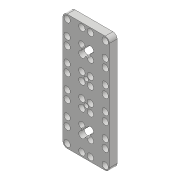
# Autodesk Inventor part: Battery_Cover
Saved by Autodesk Inventor 2018 (Build 220112000, 112)
## iProperties
Created: 2019-09-17
Part Number: Battery_Cover
Material: Generic
Document SubType Name: Modeling
Designer: Clevo
Density: 1 g/cm^3
Appearance: Default
Author: Clevo
Autodesk Inventor part; units mm, degrees
ref_plane "YZ Plane" through (0, 0, 0) normal (1, 0, 0) x (0, 1, 0)
ref_plane "XZ Plane" through (0, 0, 0) normal (0, 1, 0) x (-1, 0, 0)
ref_plane "XY Plane" through (0, 0, 0) normal (0, 0, 1) x (1, 0, 0)
sketch "Sketch1" plane through (0, 0, 0) normal (0, 1, 0) x (-1, 0, 0)
  line L0 (-22, -55) -> (22, -55)
  line L1 (22, -55) -> (22, 55)
  line L2 (22, 55) -> (-22, 55)
  line L3 (-22, 55) -> (-22, -55)
  line L4 (-22, -55) -> (22, 55) construction
  line L5 (22, -55) -> (-22, 55) construction
  point P0 (0, 0)
  dimension "d0" = 110
  dimension "d1" = 44
  constraints: 12 end point, 2 midpoint, 2 parallel, 1 horizontal, 1 perpendicular
  measures "d0" distance of L0.end L1.end
  measures "d1" distance of L1.end L2.end
extrude "Extrusion1" add sketch "Sketch1" along normal blind 7.3
sketch "Sketch2" plane through (0, 7.3, 0) normal (0, 1, 0) x (1, 0, 0)
  line L0 (22, 55) -> (-22, 55) projected
  line L1 (-22, 55) -> (-22, -55) projected
  line L2 (-22, -55) -> (22, -55) projected
  line L3 (22, -55) -> (22, 55) projected
  line L4 (0, -33) -> (-22, -33)
  line L5 (-22, -33) -> (-22, -55)
  line L6 (-22, -55) -> (0, -55)
  line L7 (0, -55) -> (0, -33)
  line L8 (0, -33) -> (-22, -55) construction
  line L9 (-22, -33) -> (0, -55) construction
  line L10 (-4, -37) -> (-18, -37)
  line L11 (-18, -37) -> (-18, -51)
  line L12 (-18, -51) -> (-4, -51)
  line L13 (-4, -51) -> (-4, -37)
  line L14 (-4, -37) -> (-18, -51) construction
  line L15 (-18, -37) -> (-4, -51) construction
  circle A0 centre (-18, -51) radius 3
  line L16 (-22, 55) -> (-22, -55) projected
  circle A1 centre (-18, -37) radius 3
  circle A2 centre (-4, -51) radius 3
  circle A3 centre (-4, -37) radius 3
  circle A4 centre (-11, -44) radius 3.75
  point P0 (0, 0)
  dimension "d4" = 22
  dimension "d5" = 22
  dimension "d6" = 14
  dimension "d7" = 7.5
  dimension "d12" = 6
  dimension "d13" = 6
  dimension "d14" = 6
  dimension "d15" = 6
  constraints: 24 end point, 5 centre point, 5 coincident, 4 midpoint, 4 parallel, 2 horizontal, 2 perpendicular, 1 point on line
  measures "d4" distance of L4.start L4.end
  measures "d5" distance of L6.end L4.start
  measures "d6" distance of L11.end L12.end
  measures "d7" diameter of A4
  measures "d12" diameter of A0
  measures "d13" diameter of A1
  measures "d14" diameter of A3
  measures "d15" diameter of A2
extrude "Extrusion2" cut sketch "Sketch2" against normal blind 7 contours A1 L11 L10 | L10 L11 A1 | A3 L13 L10 | L10 L13 A3 | A0 L12 L11 | L11 L12 A0 | A2 L12 L13 | L13 L12 A2 | A4
sketch "Sketch3" plane through (0, 0.3, 0) normal (0, 1, 0) x (1, 0, 0)
  circle A0 centre (-18, -51) radius 3 projected
  circle A1 centre (-18, -37) radius 3 projected
  circle A2 centre (-4, -51) radius 3 projected
  circle A3 centre (-4, -37) radius 3 projected
  point P0 (0, 0)
extrude "Extrusion3" cut sketch "Sketch3" against normal through all
pattern_linear "Rectangular Pattern1" count 5 spacing 22 along (0, 0, -1) count 2 spacing 22 along (1, 0, 0) of "Extrusion2", "Extrusion3"
sketch "Sketch4" plane through (0, 7.3, 0) normal (0, 1, 0) x (1, 0, 0)
  circle A0 centre (18, 51) radius 3 projected
  circle A1 centre (4, 51) radius 3 projected
  circle A2 centre (4, 37) radius 3 projected
  circle A3 centre (18, 37) radius 3 projected
  circle A4 centre (11, 44) radius 3.75 projected
  circle A5 centre (18, 29) radius 3 projected
  circle A6 centre (4, 29) radius 3 projected
  circle A7 centre (4, 15) radius 3 projected
  circle A8 centre (18, 15) radius 3 projected
  circle A9 centre (11, 22) radius 3.75 projected
  circle A10 centre (18, 7) radius 3 projected
  circle A11 centre (4, 7) radius 3 projected
  circle A12 centre (4, -7) radius 3 projected
  circle A13 centre (18, -7) radius 3 projected
  circle A14 centre (11, 0) radius 3.75 projected
  circle A15 centre (18, -15) radius 3 projected
  circle A16 centre (4, -15) radius 3 projected
  circle A17 centre (4, -29) radius 3 projected
  circle A18 centre (18, -29) radius 3 projected
  circle A19 centre (11, -22) radius 3.75 projected
  circle A20 centre (18, -37) radius 3 projected
  circle A21 centre (4, -37) radius 3 projected
  circle A22 centre (4, -51) radius 3 projected
  circle A23 centre (18, -51) radius 3 projected
  circle A24 centre (11, -44) radius 3.75 projected
  circle A25 centre (-4, 51) radius 3 projected
  circle A26 centre (-18, 51) radius 3 projected
  circle A27 centre (-18, 37) radius 3 projected
  circle A28 centre (-4, 37) radius 3 projected
  circle A29 centre (-11, 44) radius 3.75 projected
  circle A30 centre (-4, 29) radius 3 projected
  circle A31 centre (-18, 29) radius 3 projected
  circle A32 centre (-18, 15) radius 3 projected
  circle A33 centre (-4, 15) radius 3 projected
  circle A34 centre (-11, 22) radius 3.75 projected
  circle A35 centre (-4, 7) radius 3 projected
  circle A36 centre (-18, 7) radius 3 projected
  circle A37 centre (-18, -7) radius 3 projected
  circle A38 centre (-4, -7) radius 3 projected
  circle A39 centre (-11, 0) radius 3.75 projected
  circle A40 centre (-4, -15) radius 3 projected
  circle A41 centre (-18, -15) radius 3 projected
  circle A42 centre (-18, -29) radius 3 projected
  circle A43 centre (-4, -29) radius 3 projected
  circle A44 centre (-11, -22) radius 3.75 projected
  circle A45 centre (-11, -44) radius 3.75 projected
  circle A46 centre (-4, -51) radius 3 projected
  circle A47 centre (-18, -51) radius 3 projected
  circle A48 centre (-18, -37) radius 3 projected
  circle A49 centre (-4, -37) radius 3 projected
  line L0 (22, 55) -> (-22, 55) projected
  line L1 (-22, 55) -> (-22, -55) projected
  line L2 (-22, -55) -> (22, -55) projected
  line L3 (22, -55) -> (22, 55) projected
  line L4 (-16, -49) -> (16, -49)
  line L5 (16, -49) -> (16, -39)
  line L6 (16, -39) -> (-16, -39)
  line L7 (-16, -39) -> (-16, -49)
  point P0 (0, 0)
  point P1 (-16, -44)
  dimension "d22" = 10
  dimension "d23" = 5
  dimension "d24" = 5
  dimension "d25" = 5
  constraints: 8 end point, 2 parallel, 1 horizontal, 1 horizontal alignment, 1 midpoint, 1 perpendicular
  measures "d22" distance of L6.end L4.start
  measures "d23" distance from line of A45.centre L6
  measures "d24" distance from line of A45.centre L7
  measures "d25" distance from line of A24.centre L5
extrude "Extrusion4" cut sketch "Sketch4" against normal blind 2 contours L6 L5 A20 | A20 L5 A23 L4 A22 A46 A47 L7 A48 L6 A49 A21 | A21 L6 | L5 L4 A23 | A49 L6 | L4 A22 | A48 L7 L6 | L4 A46 | A47 L4 L7 picked at (15.9728, -39.1321) picked at (3.4347, -39.1582) picked at (15.9728, -48.8679) picked at (-4.5653, -39.1582) picked at (4.0602, -48.5156) picked at (-15.9728, -39.1321) picked at (-4.5653, -48.8418) picked at (-15.9728, -48.8679)
pattern_linear "Rectangular Pattern2" count 5 spacing 22 along (0, 0, -1) of "Extrusion4"
sketch "Sketch5" plane through (0, 7.3, 0) normal (0, 1, 0) x (1, 0, 0)
  line L0 (-1.7639, 49) -> (1.7639, 49) projected
  arc A0 (6.2361, 49) -> (1.7639, 49) centre (4, 51) ccw projected
  line L1 (6.2361, 49) -> (15.7639, 49) projected
  line L2 (16, 48.7639) -> (16, 39.2361) projected
  line L3 (15.7639, 39) -> (6.2361, 39) projected
  arc A1 (1.7639, 39) -> (6.2361, 39) centre (4, 37) ccw projected
  line L4 (1.7639, 39) -> (-1.7639, 39) projected
  arc A2 (-6.2361, 39) -> (-1.7639, 39) centre (-4, 37) ccw projected
  line L5 (-6.2361, 39) -> (-15.7639, 39) projected
  line L6 (-16, 39.2361) -> (-16, 48.7639) projected
  line L7 (-15.7639, 49) -> (-6.2361, 49) projected
  arc A3 (-1.7639, 49) -> (-6.2361, 49) centre (-4, 51) ccw projected
  line L8 (-1.7639, 27) -> (1.7639, 27) projected
  arc A4 (6.2361, 27) -> (1.7639, 27) centre (4, 29) ccw projected
  line L9 (6.2361, 27) -> (15.7639, 27) projected
  line L10 (16, 26.7639) -> (16, 17.2361) projected
  line L11 (15.7639, 17) -> (6.2361, 17) projected
  arc A5 (1.7639, 17) -> (6.2361, 17) centre (4, 15) ccw projected
  line L12 (1.7639, 17) -> (-1.7639, 17) projected
  arc A6 (-6.2361, 17) -> (-1.7639, 17) centre (-4, 15) ccw projected
  line L13 (-6.2361, 17) -> (-15.7639, 17) projected
  line L14 (-16, 17.2361) -> (-16, 26.7639) projected
  line L15 (-15.7639, 27) -> (-6.2361, 27) projected
  arc A7 (-1.7639, 27) -> (-6.2361, 27) centre (-4, 29) ccw projected
  line L16 (-1.7639, 5) -> (1.7639, 5) projected
  arc A8 (6.2361, 5) -> (1.7639, 5) centre (4, 7) ccw projected
  line L17 (6.2361, 5) -> (15.7639, 5) projected
  line L18 (16, 4.7639) -> (16, -4.7639) projected
  line L19 (15.7639, -5) -> (6.2361, -5) projected
  arc A9 (1.7639, -5) -> (6.2361, -5) centre (4, -7) ccw projected
  line L20 (1.7639, -5) -> (-1.7639, -5) projected
  arc A10 (-6.2361, -5) -> (-1.7639, -5) centre (-4, -7) ccw projected
  line L21 (-6.2361, -5) -> (-15.7639, -5) projected
  line L22 (-16, -4.7639) -> (-16, 4.7639) projected
  line L23 (-15.7639, 5) -> (-6.2361, 5) projected
  arc A11 (-1.7639, 5) -> (-6.2361, 5) centre (-4, 7) ccw projected
  line L24 (-1.7639, -17) -> (1.7639, -17) projected
  arc A12 (6.2361, -17) -> (1.7639, -17) centre (4, -15) ccw projected
  line L25 (6.2361, -17) -> (15.7639, -17) projected
  line L26 (16, -17.2361) -> (16, -26.7639) projected
  line L27 (15.7639, -27) -> (6.2361, -27) projected
  arc A13 (1.7639, -27) -> (6.2361, -27) centre (4, -29) ccw projected
  line L28 (1.7639, -27) -> (-1.7639, -27) projected
  arc A14 (-6.2361, -27) -> (-1.7639, -27) centre (-4, -29) ccw projected
  line L29 (-6.2361, -27) -> (-15.7639, -27) projected
  line L30 (-16, -26.7639) -> (-16, -17.2361) projected
  line L31 (-15.7639, -17) -> (-6.2361, -17) projected
  arc A15 (-1.7639, -17) -> (-6.2361, -17) centre (-4, -15) ccw projected
  line L32 (22, 55) -> (-22, 55) projected
  line L33 (-22, 55) -> (-22, -55) projected
  line L34 (-22, -55) -> (22, -55) projected
  line L35 (22, -55) -> (22, 55) projected
  arc A16 (-15.7639, -39) -> (-16, -39.2361) centre (-18, -37) ccw projected
  arc A17 (-16, -48.7639) -> (-15.7639, -49) centre (-18, -51) ccw projected
  arc A18 (-16, -26.7639) -> (-15.7639, -27) centre (-18, -29) ccw projected
  arc A19 (-15.7639, -17) -> (-16, -17.2361) centre (-18, -15) ccw projected
  arc A20 (-16, -4.7639) -> (-15.7639, -5) centre (-18, -7) ccw projected
  arc A21 (-15.7639, 5) -> (-16, 4.7639) centre (-18, 7) ccw projected
  arc A22 (-16, 17.2361) -> (-15.7639, 17) centre (-18, 15) ccw projected
  arc A23 (-15.7639, 27) -> (-16, 26.7639) centre (-18, 29) ccw projected
  arc A24 (-16, 39.2361) -> (-15.7639, 39) centre (-18, 37) ccw projected
  arc A25 (-15.7639, 49) -> (-16, 48.7639) centre (-18, 51) ccw projected
  arc A26 (15.7639, -49) -> (16, -48.7639) centre (18, -51) ccw projected
  arc A27 (16, -39.2361) -> (15.7639, -39) centre (18, -37) ccw projected
  arc A28 (15.7639, -27) -> (16, -26.7639) centre (18, -29) ccw projected
  arc A29 (16, -17.2361) -> (15.7639, -17) centre (18, -15) ccw projected
  arc A30 (15.7639, -5) -> (16, -4.7639) centre (18, -7) ccw projected
  arc A31 (16, 4.7639) -> (15.7639, 5) centre (18, 7) ccw projected
  arc A32 (15.7639, 17) -> (16, 17.2361) centre (18, 15) ccw projected
  arc A33 (16, 26.7639) -> (15.7639, 27) centre (18, 29) ccw projected
  arc A34 (15.7639, 39) -> (16, 39.2361) centre (18, 37) ccw projected
  arc A35 (16, 48.7639) -> (15.7639, 49) centre (18, 51) ccw projected
  line L36 (6.2361, -39) -> (15.7639, -39) projected
  line L37 (16, -39.2361) -> (16, -48.7639) projected
  line L38 (15.7639, -49) -> (6.2361, -49) projected
  arc A36 (1.7639, -49) -> (6.2361, -49) centre (4, -51) ccw projected
  line L39 (1.7639, -49) -> (-1.7639, -49) projected
  arc A37 (-6.2361, -49) -> (-1.7639, -49) centre (-4, -51) ccw projected
  line L40 (-6.2361, -49) -> (-15.7639, -49) projected
  line L41 (-16, -48.7639) -> (-16, -39.2361) projected
  line L42 (-15.7639, -39) -> (-6.2361, -39) projected
  arc A38 (-1.7639, -39) -> (-6.2361, -39) centre (-4, -37) ccw projected
  line L43 (-1.7639, -39) -> (1.7639, -39) projected
  arc A39 (6.2361, -39) -> (1.7639, -39) centre (4, -37) ccw projected
  circle A40 centre (-11, -44) radius 3.75 projected
  circle A41 centre (-11, 44) radius 3.75 projected
  line L44 (-6.2361, -49) -> (-16, -49) projected
  line L45 (-16, 49) -> (-6.2361, 49) projected
  line L46 (-16, -48.5) -> (-6, -48.5)
  line L47 (-6, -48.5) -> (-6, 49)
  line L48 (-6, 49) -> (-16, 49)
  line L49 (-16, 49) -> (-16, -48.5)
  point P0 (0, 0)
  point P1 (-16, 48.5)
  point P2 (-11, 49)
  constraints: 8 end point, 2 parallel, 1 horizontal, 1 midpoint, 1 perpendicular, 1 vertical alignment, 2 other
extrude "Extrusion5" cut sketch "Sketch5" against normal up to surface (2 mm away) contours L48 L47 A2 L5 A24 L49 L6 L45 L7 | L47 A7 L15 A23 L49 A24 L5 A2 | L47 A6 L13 A22 L49 L14 A23 L15 A7 | L47 A11 L23 A21 L49 A22 L13 A6 | L47 A10 L21 A20 L49 L22 A21 L23 A11 | L47 A15 L31 A19 L49 A20 L21 A10 | L47 A14 L29 A18 L49 L30 A19 L31 A15 | L47 A38 L42 A16 L49 A18 L29 A14 | L47 L46 L41 L49 A16 L42 A38 | A40 | A41
pattern_linear "Rectangular Pattern3" count 2 spacing 22 along (1, 0, 0) of "Extrusion5"
fillet "Fillet1" radius 1 47 edges at (-16, 6.3, 48.7639) (-15.7639, 6.3, 49) (-6.2361, 6.3, 49) (-1.7639, 6.3, 49) (6.2361, 6.3, 49) (15.7639, 6.3, 49) (16, 6.3, 48.7639) (16, 6.3, 39.2361) (16, 6.3, 34.7639) (16, 6.3, 31.2361) (16, 6.3, 26.7639) (16, 6.3, 17.2361) (16, 6.3, 12.7639) (16, 6.3, 9.2361) (16, 6.3, 4.7639) (16, 6.3, -4.7639) (16, 6.3, -9.2361) (16, 6.3, -12.7639) (16, 6.3, -17.2361) (16, 6.3, -26.7639) (16, 6.3, -31.2361) (16, 6.3, -34.7639) (16, 6.3, -39.2361) (16, 6.3, -48.7639) (15.7639, 6.3, -49) (6.2361, 6.3, -49) (1.7639, 6.3, -49) (-1.7639, 6.3, -49) (-6.2361, 6.3, -49) (-15.7639, 6.3, -49) (-16, 6.3, -48.7639) (-16, 6.3, -39.2361) (-16, 6.3, -34.7639) (-16, 6.3, -31.2361) (-16, 6.3, -26.7639) (-16, 6.3, -17.2361) (-16, 6.3, -12.7639) (-16, 6.3, -9.2361) (-16, 6.3, -4.7639) (-16, 6.3, 4.7639) (-16, 6.3, 9.2361) (-16, 6.3, 12.7639) (-16, 6.3, 17.2361) (-16, 6.3, 26.7639) (-16, 6.3, 31.2361) (-16, 6.3, 34.7639) (1.7639, 6.3, 49)
sketch "Sketch6" plane through (0, 7.3, 0) normal (0, 1, 0) x (1, 0, 0)
  line L0 (6, -34.7639) -> (6, -31.2361) projected
  arc A0 (1.7639, -27) -> (6, -31.2361) centre (4, -29) ccw projected
  line L1 (1.7639, -27) -> (-1.7639, -27) projected
  arc A1 (-6, -31.2361) -> (-1.7639, -27) centre (-4, -29) ccw projected
  line L2 (-6, -31.2361) -> (-6, -34.7639) projected
  arc A2 (-1.7639, -39) -> (-6, -34.7639) centre (-4, -37) ccw projected
  line L3 (-1.7639, -39) -> (1.7639, -39) projected
  arc A3 (6, -34.7639) -> (1.7639, -39) centre (4, -37) ccw projected
  circle A4 centre (0, -33) radius 4.25
  point P0 (0, 0)
  point P1 (-6, -33)
  point P2 (0, -27)
  dimension "d37" = 8.5
  constraints: 2 midpoint, 1 centre point, 1 horizontal alignment, 1 vertical alignment
  measures "d37" diameter of A4
extrude "Extrusion6" cut sketch "Sketch6" against normal through all contours A4 A3 | A3 A4 A2 A1 A0 | A0 A4 | A4 A2 | A1 A4
pattern_linear "Rectangular Pattern4" count 2 spacing 66 along (0, 0, -1) of "Extrusion6"
sketch "Sketch7" plane through (0, 7.3, 0) normal (0, 1, 0) x (1, 0, 0)
  line L0 (6, -12.7639) -> (6, -9.2361) projected
  arc A0 (1.7639, -5) -> (6, -9.2361) centre (4, -7) ccw projected
  line L1 (1.7639, -5) -> (-1.7639, -5) projected
  arc A1 (-6, -9.2361) -> (-1.7639, -5) centre (-4, -7) ccw projected
  line L2 (-6, -9.2361) -> (-6, -12.7639) projected
  arc A2 (-1.7639, -17) -> (-6, -12.7639) centre (-4, -15) ccw projected
  line L3 (-1.7639, -17) -> (1.7639, -17) projected
  arc A3 (6, -12.7639) -> (1.7639, -17) centre (4, -15) ccw projected
  circle A4 centre (0, -11) radius 2.1
  point P0 (0, 0)
  point P1 (-6, -11)
  point P2 (0, -5)
  dimension "d43" = 4.2
  constraints: 2 midpoint, 1 centre point, 1 horizontal alignment, 1 vertical alignment
  measures "d43" diameter of A4
extrude "Extrusion7" cut sketch "Sketch7" against normal through all contours A4
pattern_linear "Rectangular Pattern5" count 2 spacing 22 along (0, 0, -1) of "Extrusion7"
fillet "Fillet2" radius 4 4 edges at (22, 3.65, 55) (-22, 3.65, 55) (22, 3.65, -55) (-22, 3.65, -55)
fillet "Fillet3" radius 0.5 16 edges at (-4.13, 3.65, 31.9972) (-4.13, 3.65, 34.0028) (-1.0028, 3.65, 37.13) (1.0028, 3.65, 37.13) (1.0028, 3.65, 28.87) (-1.0028, 3.65, 28.87) (4.13, 3.65, 34.0028) (4.13, 3.65, 31.9972) (-4.13, 3.65, -34.0028) (-4.13, 3.65, -31.9972) (-1.0028, 3.65, -28.87) (1.0028, 3.65, -28.87) (-1.0028, 3.65, -37.13) (1.0028, 3.65, -37.13) (4.13, 3.65, -31.9972) (4.13, 3.65, -34.0028)
fillet "Fillet4" radius 1 10 edges at (7.25, 0.3, -44) (7.25, 0.3, -22) (7.25, 0.3, 0) (7.25, 0.3, 22) (7.25, 0.3, 44) (-14.75, 0.3, 44) (-14.75, 0.3, 22) (-14.75, 0.3, 0) (-14.75, 0.3, -22) (-14.75, 0.3, -44)
sketch "Sketch8" plane through (0, 7.3, 0) normal (0, 1, 0) x (1, 0, 0)
  arc A0 (-18, 55) -> (-22, 51) centre (-18, 51) ccw projected
  line L0 (-22, 51) -> (-22, -51) projected
  arc A1 (-22, -51) -> (-18, -55) centre (-18, -51) ccw projected
  line L1 (-18, -55) -> (18, -55) projected
  arc A2 (18, -55) -> (22, -51) centre (18, -51) ccw projected
  line L2 (22, -51) -> (22, 51) projected
  arc A3 (22, 51) -> (18, 55) centre (18, 51) ccw projected
  line L3 (18, 55) -> (-18, 55) projected
  arc A4 (1.0953, -50.25) -> (0.127, -49) centre (0.127, -50) ccw projected
  line L4 (0.127, -49) -> (-0.127, -49) projected
  arc A5 (-0.127, -49) -> (-1.0953, -50.25) centre (-0.127, -50) ccw projected
  arc A6 (-6.9047, -50.25) -> (-1.0953, -50.25) centre (-4, -51) ccw projected
  arc A7 (-6.9047, -50.25) -> (-7.873, -49) centre (-7.873, -50) ccw projected
  line L5 (-7.873, -49) -> (-14.127, -49) projected
  arc A8 (-14.127, -49) -> (-15.0953, -50.25) centre (-14.127, -50) ccw projected
  arc A9 (-17.25, -48.0953) -> (-15.0953, -50.25) centre (-18, -51) ccw projected
  arc A10 (-17.25, -48.0953) -> (-16, -47.127) centre (-17, -47.127) ccw projected
  line L6 (-16, -47.127) -> (-16, -39.2361) projected
  arc A11 (-17.25, -34.0953) -> (-16, -39.2361) centre (-18, -37) ccw projected
  arc A12 (-17.25, -34.0953) -> (-16, -33.127) centre (-17, -33.127) ccw projected
  line L7 (-16, -33.127) -> (-16, -32.873) projected
  arc A13 (-16, -32.873) -> (-17.25, -31.9047) centre (-17, -32.873) ccw projected
  arc A14 (-17.25, -26.0953) -> (-17.25, -31.9047) centre (-18, -29) ccw projected
  arc A15 (-17.25, -26.0953) -> (-16, -25.127) centre (-17, -25.127) ccw projected
  line L8 (-16, -25.127) -> (-16, -18.873) projected
  arc A16 (-16, -18.873) -> (-17.25, -17.9047) centre (-17, -18.873) ccw projected
  arc A17 (-17.25, -12.0953) -> (-17.25, -17.9047) centre (-18, -15) ccw projected
  arc A18 (-17.25, -12.0953) -> (-16, -11.127) centre (-17, -11.127) ccw projected
  line L9 (-16, -11.127) -> (-16, -10.873) projected
  arc A19 (-16, -10.873) -> (-17.25, -9.9047) centre (-17, -10.873) ccw projected
  arc A20 (-17.25, -4.0953) -> (-17.25, -9.9047) centre (-18, -7) ccw projected
  arc A21 (-17.25, -4.0953) -> (-16, -3.127) centre (-17, -3.127) ccw projected
  line L10 (-16, -3.127) -> (-16, 3.127) projected
  arc A22 (-16, 3.127) -> (-17.25, 4.0953) centre (-17, 3.127) ccw projected
  arc A23 (-17.25, 9.9047) -> (-17.25, 4.0953) centre (-18, 7) ccw projected
  arc A24 (-17.25, 9.9047) -> (-16, 10.873) centre (-17, 10.873) ccw projected
  line L11 (-16, 10.873) -> (-16, 11.127) projected
  arc A25 (-16, 11.127) -> (-17.25, 12.0953) centre (-17, 11.127) ccw projected
  arc A26 (-17.25, 17.9047) -> (-17.25, 12.0953) centre (-18, 15) ccw projected
  arc A27 (-17.25, 17.9047) -> (-16, 18.873) centre (-17, 18.873) ccw projected
  line L12 (-16, 18.873) -> (-16, 25.127) projected
  arc A28 (-16, 25.127) -> (-17.25, 26.0953) centre (-17, 25.127) ccw projected
  arc A29 (-17.25, 31.9047) -> (-17.25, 26.0953) centre (-18, 29) ccw projected
  arc A30 (-17.25, 31.9047) -> (-16, 32.873) centre (-17, 32.873) ccw projected
  line L13 (-16, 32.873) -> (-16, 33.127) projected
  arc A31 (-16, 33.127) -> (-17.25, 34.0953) centre (-17, 33.127) ccw projected
  arc A32 (-17.25, 39.9047) -> (-17.25, 34.0953) centre (-18, 37) ccw projected
  arc A33 (-17.25, 39.9047) -> (-16, 40.873) centre (-17, 40.873) ccw projected
  line L14 (-16, 40.873) -> (-16, 47.127) projected
  arc A34 (-16, 47.127) -> (-17.25, 48.0953) centre (-17, 47.127) ccw projected
  arc A35 (-15.0953, 50.25) -> (-17.25, 48.0953) centre (-18, 51) ccw projected
  arc A36 (-15.0953, 50.25) -> (-14.127, 49) centre (-14.127, 50) ccw projected
  line L15 (-14.127, 49) -> (-7.873, 49) projected
  arc A37 (-7.873, 49) -> (-6.9047, 50.25) centre (-7.873, 50) ccw projected
  arc A38 (-1.0953, 50.25) -> (-6.9047, 50.25) centre (-4, 51) ccw projected
  arc A39 (-1.0953, 50.25) -> (-0.127, 49) centre (-0.127, 50) ccw projected
  line L16 (-0.127, 49) -> (0.127, 49) projected
  arc A40 (0.127, 49) -> (1.0953, 50.25) centre (0.127, 50) ccw projected
  arc A41 (6.9047, 50.25) -> (1.0953, 50.25) centre (4, 51) ccw projected
  arc A42 (6.9047, 50.25) -> (7.873, 49) centre (7.873, 50) ccw projected
  line L17 (7.873, 49) -> (14.127, 49) projected
  arc A43 (14.127, 49) -> (15.0953, 50.25) centre (14.127, 50) ccw projected
  arc A44 (17.25, 48.0953) -> (15.0953, 50.25) centre (18, 51) ccw projected
  arc A45 (17.25, 48.0953) -> (16, 47.127) centre (17, 47.127) ccw projected
  line L18 (16, 47.127) -> (16, 40.873) projected
  arc A46 (16, 40.873) -> (17.25, 39.9047) centre (17, 40.873) ccw projected
  arc A47 (17.25, 34.0953) -> (17.25, 39.9047) centre (18, 37) ccw projected
  arc A48 (17.25, 34.0953) -> (16, 33.127) centre (17, 33.127) ccw projected
  line L19 (16, 33.127) -> (16, 32.873) projected
  arc A49 (16, 32.873) -> (17.25, 31.9047) centre (17, 32.873) ccw projected
  arc A50 (17.25, 26.0953) -> (17.25, 31.9047) centre (18, 29) ccw projected
  arc A51 (17.25, 26.0953) -> (16, 25.127) centre (17, 25.127) ccw projected
  line L20 (16, 25.127) -> (16, 18.873) projected
  arc A52 (16, 18.873) -> (17.25, 17.9047) centre (17, 18.873) ccw projected
  arc A53 (17.25, 12.0953) -> (17.25, 17.9047) centre (18, 15) ccw projected
  arc A54 (17.25, 12.0953) -> (16, 11.127) centre (17, 11.127) ccw projected
  line L21 (16, 11.127) -> (16, 10.873) projected
  arc A55 (16, 10.873) -> (17.25, 9.9047) centre (17, 10.873) ccw projected
  arc A56 (17.25, 4.0953) -> (17.25, 9.9047) centre (18, 7) ccw projected
  arc A57 (17.25, 4.0953) -> (16, 3.127) centre (17, 3.127) ccw projected
  line L22 (16, 3.127) -> (16, -3.127) projected
  arc A58 (16, -3.127) -> (17.25, -4.0953) centre (17, -3.127) ccw projected
  arc A59 (17.25, -9.9047) -> (17.25, -4.0953) centre (18, -7) ccw projected
  arc A60 (17.25, -9.9047) -> (16, -10.873) centre (17, -10.873) ccw projected
  line L23 (16, -10.873) -> (16, -11.127) projected
  arc A61 (16, -11.127) -> (17.25, -12.0953) centre (17, -11.127) ccw projected
  arc A62 (17.25, -17.9047) -> (17.25, -12.0953) centre (18, -15) ccw projected
  arc A63 (17.25, -17.9047) -> (16, -18.873) centre (17, -18.873) ccw projected
  line L24 (16, -18.873) -> (16, -25.127) projected
  arc A64 (16, -25.127) -> (17.25, -26.0953) centre (17, -25.127) ccw projected
  arc A65 (17.25, -31.9047) -> (17.25, -26.0953) centre (18, -29) ccw projected
  arc A66 (17.25, -31.9047) -> (16, -32.873) centre (17, -32.873) ccw projected
  line L25 (16, -32.873) -> (16, -33.127) projected
  arc A67 (16, -33.127) -> (17.25, -34.0953) centre (17, -33.127) ccw projected
  arc A68 (17.25, -39.9047) -> (17.25, -34.0953) centre (18, -37) ccw projected
  arc A69 (17.25, -39.9047) -> (16, -40.873) centre (17, -40.873) ccw projected
  line L26 (16, -40.873) -> (16, -47.127) projected
  arc A70 (16, -47.127) -> (17.25, -48.0953) centre (17, -47.127) ccw projected
  arc A71 (15.0953, -50.25) -> (17.25, -48.0953) centre (18, -51) ccw projected
  arc A72 (15.0953, -50.25) -> (14.127, -49) centre (14.127, -50) ccw projected
  line L27 (14.127, -49) -> (7.873, -49) projected
  arc A73 (7.873, -49) -> (6.9047, -50.25) centre (7.873, -50) ccw projected
  arc A74 (1.0953, -50.25) -> (6.9047, -50.25) centre (4, -51) ccw projected
  line L28 (18, 55) -> (-18, 55) projected
  line L29 (7.873, 49) -> (14.127, 49) projected
  line L30 (12.25, 55) -> (9.75, 55)
  line L31 (9.75, 55) -> (9.75, 49)
  line L32 (9.75, 49) -> (12.25, 49)
  line L33 (12.25, 49) -> (12.25, 55)
  circle A75 centre (11, 44) radius 3.75 projected
  point P0 (0, 0)
  point P1 (11, 49)
  dimension "d52" = 2.5
  constraints: 8 end point, 2 parallel, 2 point on line, 1 horizontal, 1 midpoint, 1 perpendicular, 1 vertical alignment
  measures "d52" distance of L31.end L32.end
extrude "Extrusion8" cut sketch "Sketch8" against normal blind 3 contours L3 L33 L17 L31
fillet "Fillet5" radius 0.5 4 edges at (12.25, 4.3, -52) (9.75, 4.3, -52) (9.75, 7.3, -52) (12.25, 7.3, -52)
equation "\"d5\" = d4"
equation "\"d13\" = d12"
equation "\"d14\" = d13"
equation "\"d15\" = d14"
equation "\"d25\" = d24"
body "Solid1"
